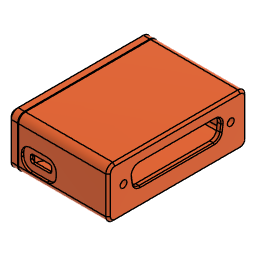
PicoBOB_Case_miniwini (Autodesk Fusion 360 design; units mm, degrees)
Autodesk Fusion 360 part; units mm, degrees
sketch "Skizze1" plane through (0, 0, 0) normal (0, 1, 0) x (1, 0, 0)
  line L0 (-0.5042, -13) -> (-0.5042, 5.2251)
  line L1 (37, -13) -> (-0.5042, -13)
  line L2 (-0.5042, 5.2251) -> (37, 5.2251)
  line L3 (37, 5.2251) -> (37, -13)
  constraint horizontal L1
  constraint vertical L0
  constraint horizontal L2
  constraint vertical L3
extrude "Extrusion1" add sketch "Skizze1" along normal blind 55 and the other way blind 2 makes body 1
sketch "Skizze2" plane through (0, -2, 0) normal (0, -1, 0) x (1, 0, 0)
  line L0 (-0.5042, -5.2251) -> (37, -5.2251)
  line L1 (37, -5.2251) -> (37, 13)
  line L2 (37, 13) -> (-0.5042, 13)
  line L3 (-0.5042, 13) -> (-0.5042, -5.2251)
  arc A0 (13.2201, 1.5046) -> (12.2201, 2.5046) centre (12.2201, 1.5046) ccw
  line L4 (13.2201, -0.0089) -> (13.2201, 1.5046)
  line L5 (12.2201, 2.5046) -> (4.9729, 2.5046)
  line L6 (3.9729, 1.5046) -> (3.9729, -0.0089)
  arc A1 (4.9729, 2.5046) -> (3.9729, 1.5046) centre (4.9729, 1.5046) ccw
  arc A2 (3.9729, -0.0089) -> (4.9729, -1.0089) centre (4.9729, -0.0089) ccw
  arc A3 (12.2201, -1.0089) -> (13.2201, -0.0089) centre (12.2201, -0.0089) ccw
  line L7 (4.9729, -1.0089) -> (12.2201, -1.0089)
  dimension "d5" = 1
  constraint horizontal L7
  constraint vertical L4
  constraint horizontal L5
  constraint vertical L6
  constraint tangent A2 L7
  constraint tangent L6 A2
  constraint tangent A3 L7
  constraint tangent L4 A3
  constraint equal A2 A3
  constraint tangent A0 L4
  constraint tangent A0 L5
  constraint equal A0 A2
  constraint tangent L5 A1
  constraint tangent L6 A1
  constraint equal A1 A2
  measures "d5" radius of A2
sketch "Skizze3" plane through (18.2479, -2, 3.8875) normal (0, -1, 0) x (1, 0, 0)
sketch "Skizze4" plane through (0, 55, 0) normal (0, 1, 0) x (-1, 0, 0)
  line L0 (-37, -5.2251) -> (0.5042, -5.2251)
  line L1 (0.5042, -5.2251) -> (0.5042, 13)
  line L2 (0.5042, 13) -> (-37, 13)
  line L3 (-37, 13) -> (-37, -5.2251)
  arc A0 (-2.7472, -1.2526) -> (-1.7472, -0.2526) centre (-2.7472, -0.2526) ccw
  line L4 (-10.2472, 1.073) -> (-10.2472, -0.2526)
  arc A1 (-1.7472, 1.073) -> (-2.7472, 2.073) centre (-2.7472, 1.073) ccw
  arc A2 (-9.2472, 2.073) -> (-10.2472, 1.073) centre (-9.2472, 1.073) ccw
  line L5 (-9.2472, -1.2526) -> (-2.7472, -1.2526)
  line L6 (-1.7472, -0.2526) -> (-1.7472, 1.073)
  line L7 (-2.7472, 2.073) -> (-9.2472, 2.073)
  arc A3 (-10.2472, -0.2526) -> (-9.2472, -1.2526) centre (-9.2472, -0.2526) ccw
  point P0 (-17, 4)
  dimension "d6" = 1
  dimension "d25" = 8.5
  constraint horizontal L5
  constraint vertical L6
  constraint horizontal L7
  constraint vertical L4
  constraint tangent L5 A3
  constraint tangent L4 A3
  constraint tangent A0 L5
  constraint tangent A0 L6
  constraint equal A0 A3
  constraint tangent A1 L6
  constraint tangent A1 L7
  constraint equal A1 A3
  constraint tangent A2 L7
  constraint tangent L4 A2
  constraint equal A2 A3
  measures "d6" radius of A3
  measures "d25" distance of L4 L6
sketch "Skizze5" plane through (-0.5042, 0, 0) normal (-1, 0, 0) x (0, -1, 0)
  line L0 (2, 13) -> (-55, 13)
  line L1 (-55, 13) -> (-55, -5.2251)
  line L2 (-55, -5.2251) -> (2, -5.2251)
  line L3 (2, -5.2251) -> (2, 13)
  circle A0 centre (-44.1519, 1.2749) radius 1.5
  circle A1 centre (-38.3789, 1.2749) radius 1.5
  dimension "d7" = 3
  dimension "d8" = 3
  dimension "d96" = 6.5
  dimension "d97" = 6.5
  measures "d7" diameter of A1
  measures "d8" diameter of A0
  measures "d96" distance of L2 A0.centre
  measures "d97" distance of L2 A1.centre
sketch "Skizze6" plane through (37, 0, 0) normal (1, 0, 0) x (0, 1, 0)
  line L0 (-2, -5.2251) -> (55, -5.2251)
  line L1 (55, -5.2251) -> (55, 13)
  line L2 (55, 13) -> (-2, 13)
  line L3 (-2, 13) -> (-2, -5.2251)
  arc A0 (42.5924, 0.85) -> (45.5632, 3.4325) centre (42.5924, 3.85) ccw
  line L4 (42.5924, 1.35) -> (10.0575, 1.35)
  arc A1 (42.5924, 1.35) -> (45.068, 3.5021) centre (42.5924, 3.85) ccw
  arc A2 (45.4756, 6.4021) -> (42.9999, 9.25) centre (42.9999, 6.75) ccw
  arc A3 (50.8749, -0.95) -> (52.8749, 1.05) centre (50.8749, 1.05) ccw
  arc A4 (52.8749, 9.55) -> (50.8749, 11.55) centre (50.8749, 9.55) ccw
  line L5 (1.7749, -0.95) -> (50.8749, -0.95)
  line L6 (50.8749, 11.55) -> (1.7749, 11.55)
  arc A5 (9.6499, 9.25) -> (7.1743, 6.4021) centre (9.6499, 6.75) ccw
  arc A6 (9.6499, 9.75) -> (6.6791, 6.3325) centre (9.6499, 6.75) ccw
  circle A7 centre (2.7749, 5.3) radius 1.5
  line L7 (42.5924, 0.85) -> (10.0575, 0.85)
  line L8 (52.8749, 1.05) -> (52.8749, 9.55)
  arc A8 (52.8749, 9.55) -> (50.8749, 11.55) centre (50.8749, 9.55) ccw
  arc A9 (7.5818, 3.5021) -> (10.0575, 1.35) centre (10.0575, 3.85) ccw
  arc A10 (-0.2251, 1.05) -> (1.7749, -0.95) centre (1.7749, 1.05) ccw
  arc A11 (9.6499, 9.25) -> (7.1743, 6.4021) centre (9.6499, 6.75) ccw
  line L9 (7.5818, 3.5021) -> (7.1743, 6.4021)
  arc A12 (7.5818, 3.5021) -> (10.0575, 1.35) centre (10.0575, 3.85) ccw
  arc A13 (1.7749, 11.55) -> (-0.2251, 9.55) centre (1.7749, 9.55) ccw
  line L10 (-0.2251, 9.55) -> (-0.2251, 1.05)
  arc A14 (-0.2251, 1.05) -> (1.7749, -0.95) centre (1.7749, 1.05) ccw
  arc A15 (7.0867, 3.4325) -> (10.0575, 0.85) centre (10.0575, 3.85) ccw
  arc A16 (1.7749, 11.55) -> (-0.2251, 9.55) centre (1.7749, 9.55) ccw
  line L11 (7.0867, 3.4325) -> (6.6791, 6.3325)
  line L12 (7.5818, 3.5021) -> (7.1743, 6.4021)
  line L13 (45.4756, 6.4021) -> (45.068, 3.5021)
  line L14 (9.6499, 9.25) -> (42.9999, 9.25)
  arc A17 (50.8749, -0.95) -> (52.8749, 1.05) centre (50.8749, 1.05) ccw
  arc A18 (45.4756, 6.4021) -> (42.9999, 9.25) centre (42.9999, 6.75) ccw
  line L15 (45.4756, 6.4021) -> (45.068, 3.5021)
  circle A19 centre (49.8749, 5.3) radius 1.5
  line L16 (52.8749, 1.05) -> (52.8749, 9.55)
  line L17 (9.6499, 9.25) -> (42.9999, 9.25)
  line L18 (45.9707, 6.3325) -> (45.5632, 3.4325)
  line L19 (-0.2251, 9.55) -> (-0.2251, 1.05)
  line L20 (42.5924, 1.35) -> (10.0575, 1.35)
  arc A20 (45.9707, 6.3325) -> (42.9999, 9.75) centre (42.9999, 6.75) ccw
  line L21 (1.7749, -0.95) -> (50.8749, -0.95)
  line L22 (9.6499, 9.75) -> (42.9999, 9.75)
  arc A21 (42.5924, 1.35) -> (45.068, 3.5021) centre (42.5924, 3.85) ccw
  line L23 (50.8749, 11.55) -> (1.7749, 11.55)
  point P0 (-1, -1)
  dimension "d9" = 0.5
  dimension "d89" = 3
  dimension "d91" = 3
  measures "d89" diameter of A7
  measures "d91" diameter of A19
shell "Schale1" thickness 2 outward yes removed faces 0 bodies 1
fillet "Abrundung1" radius 3 4 edges at (18.2479, -4, 15) (18.2479, -4, -7.2251) (18.2479, 57, -7.2251) (18.2479, 57, 15) on bodies 1
extrude "Extrusion2" cut sketch "Skizze2" along normal blind 9 and the other way blind 10 contours A0 L4 L5 L6 A1 A2 A3 L7 bodies 1
extrude "Extrusion3" cut sketch "Skizze5" along normal blind 12 contours A0 | A1 bodies 1
extrude "Extrusion4" cut sketch "Skizze4" along normal blind 16 contours A0 L4 A1 A2 L5 L6 L7 A3 bodies 1
extrude "Extrusion5" cut sketch "Skizze6" along normal blind 10 contours A0 A6 L7 A15 L11 L18 A20 L22 | L4 A1 A2 A5 A9 A11 L9 A12 L12 L13 L14 A18 L15 L17 L20 A21 | A7 | A19 bodies 1
other "Grundnetzelement1"
other "Ändern1"
fillet "Abrundung2" radius 1 4 edges at (18.2479, -2, 13) (18.2479, -2, -5.2251) (18.2479, 55, -5.2251) (18.2479, 55, 13) on bodies 1
sketch "Skizze7" plane through (0, 57, 0) normal (0, 1, 0) x (-1, 0, 0)
  line L0 (-10.2472, -0.2526) -> (-10.2472, 1.073)
  arc A0 (-9.2472, 2.073) -> (-10.2472, 1.073) centre (-9.2472, 1.073) ccw
  line L1 (-9.2472, 2.073) -> (-2.7472, 2.073)
  arc A1 (-1.7472, 1.073) -> (-2.7472, 2.073) centre (-2.7472, 1.073) ccw
  line L2 (-1.7472, 1.073) -> (-1.7472, -0.2526)
  arc A2 (-2.7472, -1.2526) -> (-1.7472, -0.2526) centre (-2.7472, -0.2526) ccw
  line L3 (-2.7472, -1.2526) -> (-9.2472, -1.2526)
  arc A3 (-10.2472, -0.2526) -> (-9.2472, -1.2526) centre (-9.2472, -0.2526) ccw
  line L4 (2.5042, 12) -> (-39, 12)
  line L5 (-39, 12) -> (-39, -4.2251)
  line L6 (-39, -4.2251) -> (2.5042, -4.2251)
  line L7 (2.5042, -4.2251) -> (2.5042, 12)
  line L8 (-1.7472, -0.2526) -> (-1.7472, 1.073)
  arc A4 (-1.7472, 1.073) -> (-2.7472, 2.073) centre (-2.7472, 1.073) ccw
  line L9 (-9.2472, -1.2526) -> (-2.7472, -1.2526)
  arc A5 (-9.2472, 2.073) -> (-10.2472, 1.073) centre (-9.2472, 1.073) ccw
  line L10 (-2.7472, 2.073) -> (-9.2472, 2.073)
  arc A6 (-2.7472, -1.2526) -> (-1.7472, -0.2526) centre (-2.7472, -0.2526) ccw
  arc A7 (-10.2472, -0.2526) -> (-9.2472, -1.2526) centre (-9.2472, -0.2526) ccw
  line L11 (-10.2472, 1.073) -> (-10.2472, -0.2526)
  arc A8 (0.2528, 1.073) -> (-2.7472, 4.073) centre (-2.7472, 1.073) ccw
  line L12 (-2.7472, 4.073) -> (-9.2472, 4.073)
  arc A9 (-9.2472, 4.073) -> (-12.2472, 1.073) centre (-9.2472, 1.073) ccw
  line L13 (-12.2472, 1.073) -> (-12.2472, -0.2526)
  arc A10 (-12.2472, -0.2526) -> (-9.2472, -3.2526) centre (-9.2472, -0.2526) ccw
  line L14 (-9.2472, -3.2526) -> (-2.7472, -3.2526)
  arc A11 (-2.7472, -3.2526) -> (0.2528, -0.2526) centre (-2.7472, -0.2526) ccw
  line L15 (0.2528, -0.2526) -> (0.2528, 1.073)
  dimension "d28" = 1
  dimension "d29" = 8.5
  dimension "d30" = 2
  constraint horizontal L9
  constraint vertical L8
  constraint horizontal L10
  constraint vertical L11
  constraint tangent L9 A7
  constraint tangent A7 L11
  constraint tangent L9 A6
  constraint tangent L8 A6
  constraint equal A6 A7
  constraint tangent L8 A4
  constraint tangent A4 L10
  constraint equal A4 A7
  constraint tangent A5 L10
  constraint tangent A5 L11
  constraint equal A5 A7
  measures "d28" radius of A7
  measures "d29" distance of L8 L11
  measures "d30" distance of A4
extrude "Extrusion6" cut sketch "Skizze7" against normal blind 1 contours L0 A0 L1 A1 L2 A2 L3 A3 L8 A4 L9 A5 L10 A6 A7 L11 | A8 L12 A9 L13 A10 L14 A11 L15 bodies 1
sketch "Skizze8" plane through (0, -4, 0) normal (0, -1, 0) x (1, 0, 0)
  arc A0 (3.9729, -0.0089) -> (4.9729, -1.0089) centre (4.9729, -0.0089) ccw
  line L0 (3.9729, -0.0089) -> (3.9729, 1.5046)
  arc A1 (4.9729, 2.5046) -> (3.9729, 1.5046) centre (4.9729, 1.5046) ccw
  line L1 (4.9729, 2.5046) -> (12.2201, 2.5046)
  arc A2 (13.2201, 1.5046) -> (12.2201, 2.5046) centre (12.2201, 1.5046) ccw
  line L2 (13.2201, 1.5046) -> (13.2201, -0.0089)
  arc A3 (12.2201, -1.0089) -> (13.2201, -0.0089) centre (12.2201, -0.0089) ccw
  line L3 (12.2201, -1.0089) -> (4.9729, -1.0089)
  line L4 (-2.5042, -4.2251) -> (39, -4.2251)
  line L5 (39, -4.2251) -> (39, 12)
  line L6 (39, 12) -> (-2.5042, 12)
  line L7 (-2.5042, 12) -> (-2.5042, -4.2251)
  line L8 (13.2201, -0.0089) -> (13.2201, 1.5046)
  arc A4 (3.9729, -0.0089) -> (4.9729, -1.0089) centre (4.9729, -0.0089) ccw
  arc A5 (12.2201, -1.0089) -> (13.2201, -0.0089) centre (12.2201, -0.0089) ccw
  arc A6 (13.2201, 1.5046) -> (12.2201, 2.5046) centre (12.2201, 1.5046) ccw
  line L9 (3.9729, 1.5046) -> (3.9729, -0.0089)
  line L10 (4.9729, -1.0089) -> (12.2201, -1.0089)
  line L11 (12.2201, 2.5046) -> (4.9729, 2.5046)
  arc A7 (4.9729, 2.5046) -> (3.9729, 1.5046) centre (4.9729, 1.5046) ccw
  line L12 (0.9729, 1.5046) -> (0.9729, -0.0089)
  arc A8 (0.9729, -0.0089) -> (4.9729, -4.0089) centre (4.9729, -0.0089) ccw
  line L13 (4.9729, -4.0089) -> (12.2201, -4.0089)
  arc A9 (12.2201, -4.0089) -> (16.2201, -0.0089) centre (12.2201, -0.0089) ccw
  line L14 (16.2201, -0.0089) -> (16.2201, 1.5046)
  arc A10 (16.2201, 1.5046) -> (12.2201, 5.5046) centre (12.2201, 1.5046) ccw
  line L15 (12.2201, 5.5046) -> (4.9729, 5.5046)
  arc A11 (4.9729, 5.5046) -> (0.9729, 1.5046) centre (4.9729, 1.5046) ccw
  dimension "d33" = 1
  dimension "d34" = 3
  constraint horizontal L10
  constraint vertical L8
  constraint horizontal L11
  constraint vertical L9
  constraint tangent A4 L10
  constraint tangent A4 L9
  constraint tangent A5 L10
  constraint tangent L8 A5
  constraint equal A4 A5
  constraint tangent L8 A6
  constraint tangent A6 L11
  constraint equal A4 A6
  constraint tangent L11 A7
  constraint tangent L9 A7
  constraint equal A4 A7
  measures "d33" radius of A4
extrude "Extrusion7" cut sketch "Skizze8" against normal blind 1 contours A0 L0 A1 L1 A2 L2 A3 L3 L8 A4 A5 A6 L9 L10 L11 A7 | L12 A8 L13 A9 L14 A10 L15 A11 bodies 1
sketch "Skizze9" plane through (39, 0, 0) normal (1, 0, 0) x (0, 1, 0)
  line L0 (7.0867, 3.4325) -> (6.6791, 6.3325)
  arc A0 (9.6499, 9.75) -> (6.6791, 6.3325) centre (9.6499, 6.75) ccw
  line L1 (9.6499, 9.75) -> (42.9999, 9.75)
  arc A1 (45.9707, 6.3325) -> (42.9999, 9.75) centre (42.9999, 6.75) ccw
  line L2 (45.9707, 6.3325) -> (45.5632, 3.4325)
  arc A2 (42.5924, 0.85) -> (45.5632, 3.4325) centre (42.5924, 3.85) ccw
  line L3 (42.5924, 0.85) -> (10.0575, 0.85)
  arc A3 (7.0867, 3.4325) -> (10.0575, 0.85) centre (10.0575, 3.85) ccw
  arc A4 (57, 12) -> (54, 15) centre (54, 12) ccw
  line L4 (54, 15) -> (-1, 15)
  arc A5 (-1, 15) -> (-4, 12) centre (-1, 12) ccw
  line L5 (-4, 12) -> (-4, -4.2251)
  arc A6 (-4, -4.2251) -> (-1, -7.2251) centre (-1, -4.2251) ccw
  line L6 (-1, -7.2251) -> (54, -7.2251)
  arc A7 (54, -7.2251) -> (57, -4.2251) centre (54, -4.2251) ccw
  line L7 (57, -4.2251) -> (57, 12)
  circle A8 centre (2.7749, 5.3) radius 1.5
  circle A9 centre (49.8749, 5.3) radius 1.5
extrude "Extrusion9" add 1 faces at (-2.5042, 11.6319, 3.0911) along direction (-1, 0, 0) blind 2 on bodies 1 bodies 1
ref_plane "Arbeitsebene1" through (-0.5042, 26.5, 3.8875) normal (-1, 0, 0) x (0, 0, 1)
split "Teilen1" by plane through (-0.5042, 26.5, 3.8875) normal (-1, 0, 0) bodies 1 makes body 2 at (-4.5042, 11.6319, 3.0911)
sketch "Skizze10" plane through (39, 0, 0) normal (1, 0, 0) x (0, 1, 0)
  line L0 (52.5, 11.5) -> (55, 11.5)
  line L1 (52.5, 6.5) -> (55, 6.5)
  line L2 (0.5, 11.5) -> (-2, 11.5)
  line L3 (0.5, 6.5) -> (-2, 6.5)
  arc A0 (0.5, 6.5) -> (0.5, 11.5) centre (0.5, 9) ccw
  arc A1 (52.5, 11.5) -> (52.5, 6.5) centre (52.5, 9) ccw
  circle A2 centre (52.5, 9) radius 1.2
  circle A3 centre (0.5, 9) radius 1.2
  line L4 (55, 11.5) -> (55, 6.5)
  line L5 (-2, 11.5) -> (-2, 6.5)
  line L6 (-2, 13) -> (55, 13)
  dimension "d44" = 2.4
  dimension "d45" = 2.4
  dimension "d49" = 1.5
  dimension "d50" = 1.5
  constraint tangent L0 A1
  constraint horizontal L0
  constraint tangent L1 A1
  constraint horizontal L1
  constraint tangent L2 A0
  constraint horizontal L2
  constraint tangent L3 A0
  constraint horizontal L3
  constraint concentric A1 A2
  constraint concentric A0 A3
  constraint perpendicular L1 L4
  constraint perpendicular L3 L5
  measures "d44" diameter of A2
  measures "d45" diameter of A3
  measures "d49" distance of L0 L6
  measures "d50" distance of L2 L6
extrude "Extrusion10" add sketch "Skizze10" along normal blind 8 from surface at -39.5042 bodies 1
sketch "Skizze11" plane through (-4.5042, 0, 0) normal (-1, 0, 0) x (0, -1, 0)
  circle A0 centre (-44.1519, 1.2749) radius 1.5
  circle A1 centre (-38.3789, 1.2749) radius 1.5
  arc A2 (-54, 15) -> (-57, 12) centre (-54, 12) ccw
  line L0 (-57, 12) -> (-57, -4.2251)
  arc A3 (-57, -4.2251) -> (-54, -7.2251) centre (-54, -4.2251) ccw
  line L1 (-54, -7.2251) -> (1, -7.2251)
  arc A4 (1, -7.2251) -> (4, -4.2251) centre (1, -4.2251) ccw
  line L2 (4, -4.2251) -> (4, 12)
  arc A5 (4, 12) -> (1, 15) centre (1, 12) ccw
  line L3 (1, 15) -> (-54, 15)
  point P0 (-52.5, 9)
  point P1 (-0.5, 9)
hole "Bohrung1" at (-4.5042, 52.5, 9) at (-4.5042, 0.5, 9) direction (1, 0, 0) diameter 3 depth 5 tip angle 118 countersink diameter 6.5 countersink angle 90 bodies 2
sketch "Skizze12" plane through (-4.5042, 0, 0) normal (-1, 0, 0) x (0, -1, 0)
  circle A0 centre (-52.5, 9) radius 3.25
  circle A1 centre (-0.5, 9) radius 3.25
  circle A2 centre (-44.1519, 1.2749) radius 1.5
  circle A3 centre (-38.3789, 1.2749) radius 1.5
  arc A4 (-54, 15) -> (-57, 12) centre (-54, 12) ccw
  line L0 (-57, 12) -> (-57, -4.2251)
  arc A5 (-57, -4.2251) -> (-54, -7.2251) centre (-54, -4.2251) ccw
  line L1 (-54, -7.2251) -> (1, -7.2251)
  arc A6 (1, -7.2251) -> (4, -4.2251) centre (1, -4.2251) ccw
  line L2 (4, -4.2251) -> (4, 12)
  arc A7 (4, 12) -> (1, 15) centre (1, 12) ccw
  line L3 (1, 15) -> (-54, 15)
  line L4 (-53.6135, -5.1002) -> (0.9935, -5.1002)
  line L5 (0.9935, -5.1002) -> (0.9935, -2.1247)
  line L6 (0.9935, -2.1247) -> (-53.6135, -2.1247)
  line L7 (-53.6135, -2.1247) -> (-53.6135, -5.1002)
  constraint horizontal L4
  constraint vertical L5
  constraint horizontal L6
  constraint vertical L7
extrude "Extrusion11" add sketch "Skizze12" against normal blind 5.7 separate body contours L4 L5 L6 L7 makes body 3
combine "Kombinieren1" operation add target body 2 tool bodies 3
move_body "Verschieben1" bodies 2 to x (1, 0, 0) y (0, 1, 0) z (0, 0, 1) at (-10, 0, 0)
fillet "Abrundung3" radius 1.25 2 edges at (-14.5042, 45.5504, 1.8173) (-14.5042, 39.7774, 1.8173) on bodies 2
sketch "Skizze13" plane through (-14.5042, 0, 0) normal (-1, 0, 0) x (0, -1, 0)
  circle A0 centre (-44.1519, 1.2749) radius 2.75
  circle A1 centre (-52.5, 9) radius 3.25
  circle A2 centre (-0.5, 9) radius 3.25
  arc A3 (-54, 15) -> (-57, 12) centre (-54, 12) ccw
  line L0 (-57, 12) -> (-57, -4.2251)
  arc A4 (-57, -4.2251) -> (-54, -7.2251) centre (-54, -4.2251) ccw
  line L1 (-54, -7.2251) -> (1, -7.2251)
  arc A5 (1, -7.2251) -> (4, -4.2251) centre (1, -4.2251) ccw
  line L2 (4, -4.2251) -> (4, 12)
  arc A6 (4, 12) -> (1, 15) centre (1, 12) ccw
  line L3 (1, 15) -> (-54, 15)
  circle A7 centre (-38.3789, 1.2749) radius 2.75
  line L4 (-49, 13) -> (-5, 13)
  line L5 (-5, 13) -> (-5, 11)
  line L6 (-5, 11) -> (-49, 11)
  line L7 (-49, 11) -> (-49, 13)
  constraint horizontal L4
  constraint vertical L5
  constraint horizontal L6
  constraint vertical L7
extrude "Extrusion12" add sketch "Skizze13" against normal blind 13 contours L4 L5 L6 L7 bodies 2
fillet "Abrundung4" radius 5.5 2 edges at (-1.5042, 49, 12) (-1.5042, 5, 12) on bodies 2
move_body "Verschieben2" bodies 2 to x (1, 0, 0) y (0, 1, 0) z (0, 0, 1) at (10, 0, 0)
revolve "Drehen1" add 1 faces at (7.4958, -1.5667, 9) angle 90 about axis through (7.4958, -2, 6.5) along (0, 0, -1) on bodies 1 bodies 1
revolve "Drehen2" add 1 faces at (7.4958, 54.5667, 9) angle 90 about axis through (7.4958, 55, 11.5) along (0, 0, 1) on bodies 1 bodies 1
fillet "Abrundung5" radius 0.4 3 edges at (4.7458, 55, 11.5) (12.4958, 55, 9) (4.7458, 55, 6.5) on bodies 1
fillet "Abrundung6" radius 0.4 3 edges at (4.7458, -2, 6.5) (12.4958, -2, 9) (4.7458, -2, 11.5) on bodies 1
chamfer "Fase2" distance 1 angle 45 8 edges at (-4.5042, 26.5, 15) (-4.5042, 56.1213, 14.1213) (-4.5042, 57, 3.8875) (-4.5042, 56.1213, -6.3464) (-4.5042, 26.5, -7.2251) (-4.5042, -3.1213, -6.3464) (-4.5042, -4, 3.8875) (-4.5042, -3.1213, 14.1213) on bodies 2
chamfer "Fase3" distance 1 angle 45 8 edges at (39, 26.5, 15) (39, 56.1213, 14.1213) (39, 57, 3.8875) (39, 56.1213, -6.3464) (39, 26.5, -7.2251) (39, -3.1213, -6.3464) (39, -4, 3.8875) (39, -3.1213, 14.1213) on bodies 1
sketch "Skizze16" plane through (-4.5042, 0, 0) normal (-1, 0, 0) x (0, -1, 0)
  circle A0 centre (-38.3789, 1.2749) radius 2.75
  circle A1 centre (-0.5, 9) radius 3.25
  circle A2 centre (-52.5, 9) radius 3.25
  circle A3 centre (-44.1519, 1.2749) radius 2.75
  line L0 (1, 14) -> (-54, 14)
  arc A4 (-54, 14) -> (-56, 12) centre (-54, 12) ccw
  line L1 (-56, 12) -> (-56, -4.2251)
  arc A5 (-56, -4.2251) -> (-54, -6.2251) centre (-54, -4.2251) ccw
  line L2 (-54, -6.2251) -> (1, -6.2251)
  arc A6 (1, -6.2251) -> (3, -4.2251) centre (1, -4.2251) ccw
  line L3 (3, -4.2251) -> (3, 12)
  arc A7 (3, 12) -> (1, 14) centre (1, 12) ccw
  line L4 (-28.3426, -2.1247) -> (-6.0234, -2.1247)
  line L5 (-6.0234, -2.1247) -> (-6.0234, -5.1002)
  line L6 (-6.0234, -5.1002) -> (-28.3426, -5.1002)
  line L7 (-28.3426, -5.1002) -> (-28.3426, -2.1247)
  line L8 (-45.668, -2.1247) -> (-35.668, -2.1247)
  line L9 (-35.668, -2.1247) -> (-35.668, -5.1002)
  line L10 (-35.668, -5.1002) -> (-45.668, -5.1002)
  line L11 (-45.668, -5.1002) -> (-45.668, -2.1247)
  line L12 (0.9935, -2.1247) -> (-53.6135, -2.1247)
  line L13 (-53.6135, -5.1002) -> (0.9935, -5.1002)
  dimension "d77" = 10
  constraint horizontal L4
  constraint vertical L5
  constraint horizontal L6
  constraint vertical L7
  constraint horizontal L8
  constraint vertical L9
  constraint horizontal L10
  constraint vertical L11
  constraint collinear L8 L12
  constraint collinear L10 L13
  constraint collinear L4 L12
  constraint collinear L6 L13
  measures "d77" distance of L9 L11
extrude "Extrusion14" add sketch "Skizze16" against normal blind 18 from surface at -1 contours L4 L5 L6 L7 L12 L13 | L8 L9 L10 L11 L12 L13 bodies 2
fillet "Abrundung7" radius 3.5 4 edges at (14.4958, 45.668, -3.6125) (14.4958, 35.668, -3.6125) (14.4958, 28.3426, -3.6125) (14.4958, 6.0234, -3.6125) on bodies 2
fillet "Abrundung8" radius 4.5 2 edges at (1.1958, 6.0234, -3.6125) (1.1958, 45.668, -3.6125) on bodies 2
chamfer "Fase4" distance 1.6 angle 45 1 edges at (1.1958, -0.9935, -3.6125) on bodies 2
chamfer "Fase4" distance 1.6 angle 45 1 edges at (1.1958, 53.6135, -3.6125) on bodies 2
chamfer "Fase5" distance 0.2 angle 45 8 edges at (-0.5042, 26.5, 15) (-0.5042, 56.1213, 14.1213) (-0.5042, 57, 3.8875) (-0.5042, 56.1213, -6.3464) (-0.5042, 26.5, -7.2251) (-0.5042, -3.1213, -6.3464) (-0.5042, -4, 3.8875) (-0.5042, -3.1213, 14.1213) on bodies 1
chamfer "Fase6" distance 0.2 angle 45 8 edges at (-0.5042, 56.1213, 14.1213) (-0.5042, 57, 3.8875) (-0.5042, 56.1213, -6.3464) (-0.5042, 26.5, -7.2251) (-0.5042, -3.1213, -6.3464) (-0.5042, -4, 3.8875) (-0.5042, -3.1213, 14.1213) (-0.5042, 26.5, 15) on bodies 2
chamfer "Fase7" distance 0.5 angle 45 8 edges at (39, 26.3249, 9.75) (39, 45.2641, 8.7182) (39, 45.767, 4.8825) (39, 44.5606, 1.5859) (39, 26.3249, 0.85) (39, 8.0893, 1.5859) (39, 6.8829, 4.8825) (39, 7.3858, 8.7182) on bodies 1
named bodies: "PicoBob_1"
